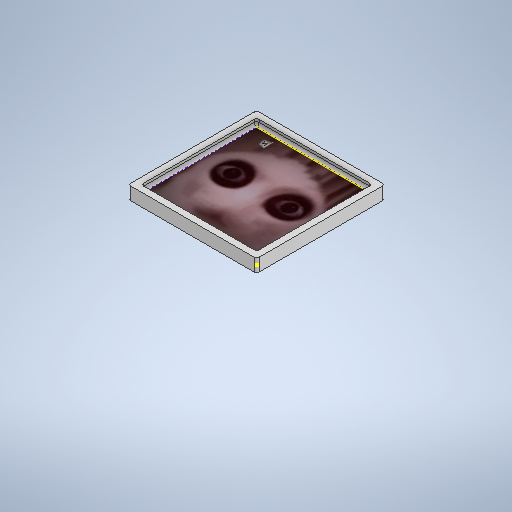
# Autodesk Inventor part: plateau
Saved by Autodesk Inventor 2025 (Build 290162010, 162A)
## iProperties
Created: 2025-02-16
Part Number: plateau
Material: Générique
Document SubType Name: Modeling
Designer: arthu
Density: 1 g/cm^3
Appearance: Par défaut
Author: arthu
Autodesk Inventor part; units mm, degrees
ref_plane "YZ Plane" through (0, 0, 0) normal (1, 0, 0) x (0, 1, 0)
ref_plane "XZ Plane" through (0, 0, 0) normal (0, 1, 0) x (-1, 0, 0)
ref_plane "XY Plane" through (0, 0, 0) normal (0, 0, 1) x (1, 0, 0)
sketch "Esquisse1" plane through (0, 0, 0) normal (0, 1, 0) x (-1, 0, 0)
  line L0 (0, 0) -> (100, 0)
  line L1 (100, 0) -> (100, -100)
  line L2 (100, -100) -> (0, -100)
  line L3 (0, -100) -> (0, 0)
  dimension "d0" = 100
  dimension "d1" = 100
  constraints: 8 end point, 2 parallel, 1 horizontal, 1 perpendicular
  measures "d0" distance of L1.end L2.end
  measures "d1" distance of L0.end L1.end
extrude "Extrusion1" add sketch "Esquisse1" along normal blind 10
sketch "Esquisse3" plane through (0, 0, 0) normal (0, -1, 0) x (1, 0, 0)
  line L0 (0, -100) -> (-100, -100) projected
  line L1 (0, -100) -> (-4.9999, -95)
  circle A0 centre (-4.9999, -95) radius 1.6952
  point P0 (0, 0)
  dimension "d4" = 7.071
  constraints: 2 end point, 1 centre point, 1 coincident
  measures "d4" distance of L0.start L1.end
hole "Perçage1" at (-4.9999, 0, -95) direction (0, 1, 0) diameter 4.9587 depth 5 thread size "M5.5x0.5" class "6H" standard "ISO Metric profile"
pattern_linear "Réseau rectangulaire1" count 2 spacing 90 along (0, 0, 1) count 2 spacing 90 along (-1, 0, 0) of "Perçage1"
fillet "Congé1" radius 2 4 edges at (0, 5, 0) (-100, 5, 0) (-100, 5, -100) (0, 5, -100)
sketch "Esquisse4" plane through (0, 10, 0) normal (0, 1, 0) x (1, 0, 0)
  circle A0 centre (-94.9999, 5) radius 2.4794 projected
  circle A1 centre (-4.9999, 95) radius 2.4794 projected
  line L0 (-94.9999, 5) -> (-4.9999, 5)
  line L1 (-4.9999, 5) -> (-4.9999, 95)
  line L2 (-4.9999, 95) -> (-94.9999, 95)
  line L3 (-94.9999, 95) -> (-94.9999, 5)
  point P0 (0, 0)
  constraints: 8 end point, 2 parallel, 1 horizontal, 1 perpendicular
extrude "Extrusion2" cut sketch "Esquisse4" against normal blind 4 contours L0 L3 A0 | A0 L3 L2 A1 L1 L0 | A1 L2 L1 picked at (-94.4574, 6.5504) picked at (-6.5503, 94.4575)
fillet "Congé2" radius 2 8 edges at (-4.9999, 8, -95) (-49.9999, 6, -95) (-94.9999, 8, -95) (-94.9999, 6, -50) (-4.9999, 6, -50) (-4.9999, 8, -5) (-49.9999, 6, -5) (-94.9999, 8, -5)
sketch "Esquisse6" plane through (0, 6, 0) normal (0, 1, 0) x (1, 0, 0)
  line L0 (-92.9999, 93) -> (-6.9999, 93) projected
  line L1 (-92.9999, 93) -> (-7.0674, 93) construction
  line L2 (-7.0674, 93) -> (-7.0674, 6.1315) construction
  line L3 (-7.0674, 6.1315) -> (-92.9999, 6.1315) construction
  line L4 (-92.9999, 6.1315) -> (-92.9999, 93) construction
  point P0 (0, 0)
  constraints: 2 other
